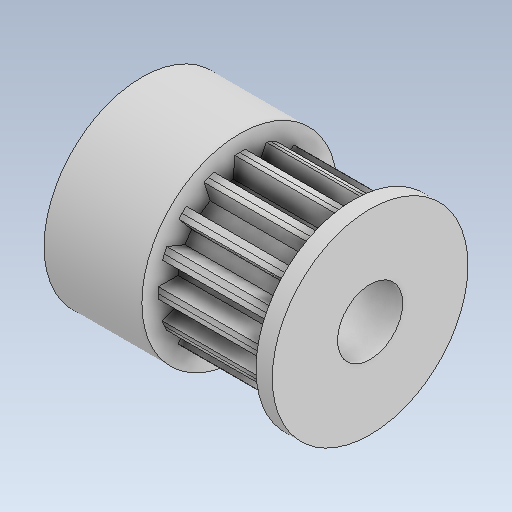
# Autodesk Inventor part: gear_16
Saved by Autodesk Inventor 2020 (Build 240168000, 168)
## iProperties
Created: 2024-02-19
Part Number: gear_16
Material: Типовые
Document SubType Name: Modeling
Designer: 4s
Density: 1 g/cm^3
Appearance: По умолчанию
Author: 4s
Autodesk Inventor part; units mm, degrees
ref_plane "YZ Plane" through (0, 0, 0) normal (1, 0, 0) x (0, 1, 0)
ref_plane "XZ Plane" through (0, 0, 0) normal (0, 1, 0) x (-1, 0, 0)
ref_plane "XY Plane" through (0, 0, 0) normal (0, 0, 1) x (1, 0, 0)
sketch "Эскиз1" plane through (0, 0, 0) normal (1, 0, 0) x (0, 1, 0)
  circle A0 centre (0, 0) radius 5
  dimension "d0" = 10
  constraints: 1 centre point, 1 coincident
  measures "d0" diameter of A0
extrude "Выдавливание1" add sketch "Эскиз1" along normal blind 7
sketch "Эскиз2" plane through (7, 0, 0) normal (1, 0, 0) x (0, 0, -1)
  circle A0 centre (0, 0) radius 6
  dimension "d3" = 12
  constraints: 1 centre point, 1 coincident
  measures "d3" diameter of A0
extrude "Выдавливание2" add sketch "Эскиз2" along normal blind 1
sketch "Эскиз3" plane through (0, 0, 0) normal (-1, 0, 0) x (0, 0, 1)
  circle A0 centre (0, 0) radius 6
  dimension "d6" = 12
  constraints: 1 centre point, 1 coincident
  measures "d6" diameter of A0
extrude "Выдавливание3" add sketch "Эскиз3" along normal blind 6
sketch "Эскиз4" plane through (8, 0, 0) normal (1, 0, 0) x (0, 0, -1)
  circle A0 centre (0, 0) radius 2
  dimension "d9" = 4
  constraints: 1 centre point, 1 coincident
  measures "d9" diameter of A0
extrude "Выдавливание4" cut sketch "Эскиз4" against normal blind 60
sketch "Эскиз5" plane through (0, 0, 0) normal (1, 0, 0) x (0, 0, -1)
  circle A0 centre (0, 0) radius 5 construction
  circle A1 centre (0, 0) radius 5 construction
  circle A2 centre (0, 0) radius 6 construction
  circle A3 centre (0, 0) radius 6 construction
  circle A4 centre (0, 0) radius 2 construction
  circle A5 centre (0, 0) radius 2 construction
  line L0 (0, 0) -> (0, 5) construction
  line L1 (0, 0) -> (1.9134, 4.6194) construction
  circle A6 centre (0, 0) radius 3.8 construction
  line L2 (0.3593, 4.9871) -> (0.3593, 3.783)
  line L3 (0.3593, 3.783) -> (1.0804, 3.6432)
  line L4 (1.0804, 3.6432) -> (1.6376, 4.7242)
  line L5 (0, 5) -> (0.3593, 4.9871)
  line L6 (1.6376, 4.7242) -> (1.9134, 4.6194)
  line L7 (-1.5765, 4.745) -> (-1.1157, 3.6325)
  line L8 (-1.1157, 3.6325) -> (-0.3961, 3.7793)
  line L9 (-0.3961, 3.7793) -> (-0.295, 4.9913)
  line L10 (-1.9134, 4.6194) -> (-1.5765, 4.745)
  line L11 (-0.295, 4.9913) -> (0, 5)
  line L12 (-3.2723, 3.7805) -> (-2.4209, 2.929)
  line L13 (-2.4209, 2.929) -> (-1.8122, 3.3401)
  line L14 (-1.8122, 3.3401) -> (-2.1826, 4.4985)
  line L15 (-3.5355, 3.5355) -> (-3.2723, 3.7805)
  line L16 (-2.1826, 4.4985) -> (-1.9134, 4.6194)
  line L17 (-4.47, 2.2404) -> (-3.3575, 1.7796)
  line L18 (-3.3575, 1.7796) -> (-2.9524, 2.3923)
  line L19 (-2.9524, 2.3923) -> (-3.738, 3.3208)
  line L20 (-4.6194, 1.9134) -> (-4.47, 2.2404)
  line L21 (-3.738, 3.3208) -> (-3.5355, 3.5355)
  line L22 (-4.9871, 0.3593) -> (-3.783, 0.3593)
  line L23 (-3.783, 0.3593) -> (-3.6432, 1.0804)
  line L24 (-3.6432, 1.0804) -> (-4.7242, 1.6376)
  line L25 (-5, 0) -> (-4.9871, 0.3593)
  line L26 (-4.7242, 1.6376) -> (-4.6194, 1.9134)
  line L27 (-4.745, -1.5765) -> (-3.6325, -1.1157)
  line L28 (-3.6325, -1.1157) -> (-3.7793, -0.3961)
  line L29 (-3.7793, -0.3961) -> (-4.9913, -0.295)
  line L30 (-4.6194, -1.9134) -> (-4.745, -1.5765)
  line L31 (-4.9913, -0.295) -> (-5, 0)
  line L32 (-3.7805, -3.2723) -> (-2.929, -2.4209)
  line L33 (-2.929, -2.4209) -> (-3.3401, -1.8122)
  line L34 (-3.3401, -1.8122) -> (-4.4985, -2.1826)
  line L35 (-3.5355, -3.5355) -> (-3.7805, -3.2723)
  line L36 (-4.4985, -2.1826) -> (-4.6194, -1.9134)
  line L37 (-2.2404, -4.47) -> (-1.7796, -3.3575)
  line L38 (-1.7796, -3.3575) -> (-2.3923, -2.9524)
  line L39 (-2.3923, -2.9524) -> (-3.3208, -3.738)
  line L40 (-1.9134, -4.6194) -> (-2.2404, -4.47)
  line L41 (-3.3208, -3.738) -> (-3.5355, -3.5355)
  line L42 (-0.3593, -4.9871) -> (-0.3593, -3.783)
  line L43 (-0.3593, -3.783) -> (-1.0804, -3.6432)
  line L44 (-1.0804, -3.6432) -> (-1.6376, -4.7242)
  line L45 (0, -5) -> (-0.3593, -4.9871)
  line L46 (-1.6376, -4.7242) -> (-1.9134, -4.6194)
  line L47 (1.5765, -4.745) -> (1.1157, -3.6325)
  line L48 (1.1157, -3.6325) -> (0.3961, -3.7793)
  line L49 (0.3961, -3.7793) -> (0.295, -4.9913)
  line L50 (1.9134, -4.6194) -> (1.5765, -4.745)
  line L51 (0.295, -4.9913) -> (0, -5)
  line L52 (3.2723, -3.7805) -> (2.4209, -2.929)
  line L53 (2.4209, -2.929) -> (1.8122, -3.3401)
  line L54 (1.8122, -3.3401) -> (2.1826, -4.4985)
  line L55 (3.5355, -3.5355) -> (3.2723, -3.7805)
  line L56 (2.1826, -4.4985) -> (1.9134, -4.6194)
  line L57 (4.47, -2.2404) -> (3.3575, -1.7796)
  line L58 (3.3575, -1.7796) -> (2.9524, -2.3923)
  line L59 (2.9524, -2.3923) -> (3.738, -3.3208)
  line L60 (4.6194, -1.9134) -> (4.47, -2.2404)
  line L61 (3.738, -3.3208) -> (3.5355, -3.5355)
  line L62 (4.9871, -0.3593) -> (3.783, -0.3593)
  line L63 (3.783, -0.3593) -> (3.6432, -1.0804)
  line L64 (3.6432, -1.0804) -> (4.7242, -1.6376)
  line L65 (5, 0) -> (4.9871, -0.3593)
  line L66 (4.7242, -1.6376) -> (4.6194, -1.9134)
  line L67 (4.745, 1.5765) -> (3.6325, 1.1157)
  line L68 (3.6325, 1.1157) -> (3.7793, 0.3961)
  line L69 (3.7793, 0.3961) -> (4.9913, 0.295)
  line L70 (4.6194, 1.9134) -> (4.745, 1.5765)
  line L71 (4.9913, 0.295) -> (5, 0)
  line L72 (3.7805, 3.2723) -> (2.929, 2.4209)
  line L73 (2.929, 2.4209) -> (3.3401, 1.8122)
  line L74 (3.3401, 1.8122) -> (4.4985, 2.1826)
  line L75 (3.5355, 3.5355) -> (3.7805, 3.2723)
  line L76 (4.4985, 2.1826) -> (4.6194, 1.9134)
  line L77 (2.2404, 4.47) -> (1.7796, 3.3575)
  line L78 (1.7796, 3.3575) -> (2.3923, 2.9524)
  line L79 (2.3923, 2.9524) -> (3.3208, 3.738)
  line L80 (1.9134, 4.6194) -> (2.2404, 4.47)
  line L81 (3.3208, 3.738) -> (3.5355, 3.5355)
  circle A7 centre (0, 0) radius 5.4727
  dimension "d12" = 22.5
  dimension "d13" = 7.6
  dimension "d16" = 360
  constraints: 164 end point, 6 point on circle, 2 centre point, 2 coincident, 1 vertical, 177 other
  measures "d12" angle of L0 L1
  measures "d13" diameter of A6
extrude "Выдавливание5" cut sketch "Эскиз5" along normal blind 7
